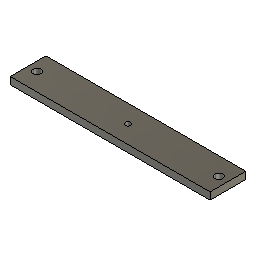
LabjackT4_railmount v2 (Autodesk Fusion 360 design; units mm, degrees)
Autodesk Fusion 360 part; units mm, degrees
note: some values were not read from the file. Set by a fixed rule: the direction of a hole.
sketch "Sketch1" plane through (0, 0, 0) normal (0, 0, 1) x (1, 0, 0)
  line L0 (0, 0) -> (139.7, 0)
  line L1 (139.7, 0) -> (139.7, 25)
  line L2 (139.7, 25) -> (0, 25)
  line L3 (0, 25) -> (0, 0)
  dimension "d1" = 139.7
  dimension "d2" = 25
  constraint horizontal L0
  constraint vertical L1
  constraint horizontal L2
  constraint vertical L3
  constraint coincident L0.start L3.end
  measures "d1" distance of L0.start L0.end
  measures "d2" distance of L0.start L2.end
extrude "Extrude1" add sketch "Sketch1" along normal blind 5
sketch "Sketch2" plane through (0, 0, 0) normal (0, 0, 1) x (1, 0, 0)
  point P0 (6.35, 12.5)
  point P1 (133.35, 12.5)
  constraint horizontal P0 P1
hole "Hole1" at (6.35, 12.5, 0) at (133.35, 12.5, 0) direction (0, 0, 1) diameter 5.5 depth 13 tip angle 118 counterbore diameter 9.1 counterbore depth 1
sketch "Sketch5" plane through (0, 0, 0) normal (0, 0, -1) x (1, 0, 0)
  circle A0 centre (6.35, -12.5) radius 4.55
  circle A1 centre (133.35, -12.5) radius 4.55
  line L0 (0, 0) -> (0, -25)
  line L1 (0, -25) -> (139.7, -25)
  line L2 (139.7, -25) -> (139.7, 0)
  line L3 (139.7, 0) -> (0, 0)
  point P0 (69.85, -12.5)
hole "Hole4" at (69.85, 12.5, 0) direction (0, 0, 1) diameter 3.75 depth 15 tip angle 118
